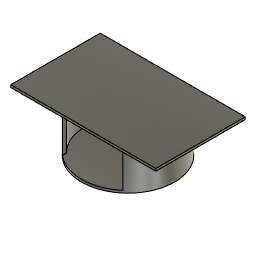
v01.00-sim-dash-g920-mount (Autodesk Fusion 360 design; units mm, degrees)
Autodesk Fusion 360 part; units mm, degrees
sketch "Sketch1" plane through (0, 0, 0) normal (0, 0, 1) x (1, 0, 0)
  circle A0 centre (0, 0) radius 38.5
  dimension "d5" = 77
  constraint coincident A0.centre origin
  measures "d5" diameter of A0
extrude "Extrude1" add sketch "Sketch1" along normal blind 2
sketch "Sketch4" plane through (0, 0, 2) normal (0, 0, 1) x (-1, 0, 0)
  circle A0 centre (0, 0) radius 38.5
  circle A1 centre (0, 0) radius 36
  circle A2 centre (0, 0) radius 38.5
  dimension "d7" = 77
  dimension "d8" = 72
  constraint concentric A0 A1
  constraint concentric A1 A2
  measures "d7" diameter of A2
  measures "d8" diameter of A1
extrude "Extrude3" add sketch "Sketch4" along normal blind 35
sketch "Sketch6" plane through (0, 0, 37) normal (0, 0, 1) x (-1, 0, 0)
  circle A0 centre (0, 0) radius 36
  circle A1 centre (0, 0) radius 38.5
  line L0 (25, -40.1842) -> (-25, -40.1842)
  line L1 (-25, -40.1842) -> (-25, 39.8158)
  line L2 (-25, 39.8158) -> (25, 39.8158)
  line L3 (25, 39.8158) -> (25, -40.1842)
  dimension "d11" = 50
  dimension "d12" = 80
  dimension "d13" = 25
  constraint horizontal L0
  constraint vertical L1
  constraint horizontal L2
  constraint vertical L3
  measures "d11" distance of L0.start L0.end
  measures "d12" distance of L0.start L2.end
  measures "d13" distance of A0.centre L3
extrude "Extrude4" cut sketch "Sketch6" against normal blind 35 contours A0 A1 L1 L3 | A0 A1 L1 L3
sketch "Sketch7" plane through (0, 0, 37) normal (0, 0, 1) x (-1, 0, 0)
  line L0 (25, 29.2788) -> (25, 25.9037)
  arc A0 (25, -25.9037) -> (25, 25.9037) centre (0, 0) ccw
  line L1 (25, -25.9037) -> (25, -29.2788)
  arc A1 (25, -29.2788) -> (25, 29.2788) centre (0, 0) ccw
  line L2 (60, -37) -> (-60, -37)
  line L3 (-60, -37) -> (-60, 37)
  line L4 (-60, 37) -> (60, 37)
  line L5 (60, 37) -> (60, -37)
  dimension "d16" = 74
  dimension "d17" = 120
  dimension "d18" = 60
  dimension "d19" = 37
  constraint horizontal L2
  constraint vertical L3
  constraint horizontal L4
  constraint vertical L5
  measures "d16" distance of L2.end L3.end
  measures "d17" distance of L2.start L2.end
  measures "d18" distance of A0.centre L5
  measures "d19" distance of A0.centre L4
extrude "Extrude5" add sketch "Sketch7" along normal blind 2 contours L0 A0 L1 A1 | L2 L3 L4 L5
